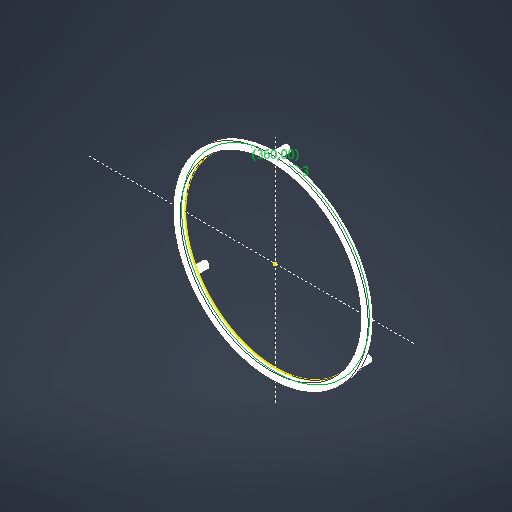
# Autodesk Inventor part: Anillo medidor
Saved by Autodesk Inventor 2026.2 (Build 302298000, 298)
## iProperties
Created: 2025-12-31
Part Number: Anillo medidor
Material: Genérico
Document SubType Name: Modeling
Designer: vicho
Density: 1 g/cm^3
Appearance: Valor por defecto
Author: vicho
Autodesk Inventor part; units mm, degrees
ref_plane "YZ Plane" through (0, 0, 0) normal (1, 0, 0) x (0, 1, 0)
ref_plane "XZ Plane" through (0, 0, 0) normal (0, 1, 0) x (-1, 0, 0)
ref_plane "XY Plane" through (0, 0, 0) normal (0, 0, 1) x (1, 0, 0)
sketch "Boceto1" plane through (0, 0, 0) normal (0, 0, 1) x (1, 0, 0)
  line L0 (0, 45.257) -> (0, -55.794) construction
  line L1 (-63.6876, 0) -> (64.1807, 0) construction
  circle A0 centre (0, 0) radius 40
  dimension "d0" = 80
  constraints: 4 end point, 2 horizontal, 2 point on line, 2 vertical, 1 centre point, 1 coincident
  measures "d0" diameter of A0
extrude "Extrusión1" add sketch "Boceto1" along normal blind 2
sketch "Boceto2" plane through (0, 0, 0) normal (0, 0, -1) x (-1, 0, 0)
  point P0 (0, 0)
shell "Vaciado1" thickness 3 removed faces 2 at (-12.1058, -2.3153, 0) at (-12.1058, -2.3153, 2)
sketch "Boceto3" plane through (0, 0, 0) normal (0, 0, -1) x (-1, 0, 0)
  circle A0 centre (0, 38.5) radius 1.5
  circle A1 centre (0, 0) radius 37 projected
  line L0 (0, 44.6838) -> (0, -50.1567) construction
  line L1 (-57.4569, 0) -> (76.4251, 0) construction
  circle A2 centre (-33.342, -19.25) radius 1.5
  circle A3 centre (33.342, -19.25) radius 1.5
  dimension "d4" = 3
  dimension "d7" = 360
  constraints: 4 end point, 3 centre point, 3 point on line, 2 horizontal, 2 vertical, 1 tangent, 7 other
  measures "d4" diameter of A0
extrude "Extrusión2" add sketch "Boceto3" along normal blind 5 contours A0 | A3 | A2
sketch "Boceto4" plane through (0, 0, 0) normal (0, 0, -1) x (-1, 0, 0)
  point P0 (0, 0)
